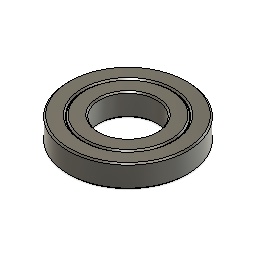
LR2051-822 (Autodesk Fusion 360 design; units mm, degrees)
Autodesk Fusion 360 part; units mm, degrees
sketch "profile" plane through (0, 0, 0) normal (0, 0, 1) x (1, 0, 0) in component "LR2051-822"
  line L0 (0, 0) -> (0, 8) construction
  line L1 (-10, 8) -> (-21, 8)
  line L2 (-21, 8) -> (-21, 0)
  line L3 (-21, 0) -> (-10, 0)
  line L4 (-10, 8) -> (-10, 0)
  line L5 (0, 8) -> (-10, 8) construction
  line L6 (-10, 0) -> (0, 0) construction
  line L7 (-15.5, 0) -> (-15.5, 1) construction
  line L8 (-15.5, 1) -> (-17, 2.5) construction
  line L9 (-17, 2.5) -> (-14, 5.5) construction
  line L10 (-14, 5.5) -> (-15.5, 7) construction
  line L11 (-15.5, 7) -> (-15.5, 8) construction
  line L12 (-10, 4) -> (-21, 4) construction
  line L13 (-15.5, 7) -> (-15.5, 1) construction
  line L14 (-15.4, 0) -> (-15.4, 1.0414)
  line L15 (-15.4, 1.0414) -> (-16.8586, 2.5)
  line L16 (-16.8586, 2.5) -> (-13.8586, 5.5)
  line L17 (-13.8586, 5.5) -> (-15.4, 7.0414)
  line L18 (-15.4, 7.0414) -> (-15.4, 8)
  line L19 (-15.6, 0) -> (-15.6, 0.9586)
  line L20 (-15.6, 0.9586) -> (-17.1414, 2.5)
  line L21 (-17.1414, 2.5) -> (-14.1414, 5.5)
  line L22 (-14.1414, 5.5) -> (-15.6, 6.9586)
  line L23 (-15.6, 6.9586) -> (-15.6, 8)
  point P0 (-15.5, 4)
  dimension "d4" = 21
  dimension "d5" = 10
  dimension "d6" = 45
  dimension "d7" = 1.5
  dimension "d8" = 1.5
  dimension "d9" = 8
  dimension "d10" = 0.1
  dimension "d11" = -0.1
  constraint coincident L0.start L6.end
  constraint vertical L0
  constraint perpendicular L0 L1
  constraint perpendicular L1 L2
  constraint perpendicular L0 L3
  constraint perpendicular L3 L4
  constraint perpendicular L0 L5
  constraint perpendicular L0 L6
  constraint midpoint L3 L7.start
  constraint perpendicular L3 L7
  constraint midpoint L1 L11.end
  constraint perpendicular L1 L11
  constraint midpoint L4 L12.start
  constraint midpoint L2 L12.end
  constraint parallel L8 L10
  constraint perpendicular L8 L9
  constraint midpoint L12 P0
  constraint coincident L9 P0
  measures "d4" distance of L2 L0.start
  measures "d5" distance of L0.start L4
  measures "d6" angle of L8 L13
  measures "d7" distance of L9.end L13
  measures "d8" distance of L8.end L11
  measures "d9" distance of L1.end L2.end
revolve "Revolve1" add sketch "profile" angle 360 about axis through (0, 0, 0) along (0, 1, 0) contours L1 L3 L4 L14 L15 L16 L17 L18 makes body 1 in component "Inner Shell"
revolve "Revolve1'" add sketch "profile" angle 360 about axis through (0, 0, 0) along (0, 1, 0) separate body contours L1 L2 L3 L19 L20 L21 L22 L23 makes body 2 in component "Outer Shell"
chamfer "Chamfer1" distance 0.5 angle 45 2 edges at (-14.3578, 8, 5.5689) (-14.3578, 0, 5.5689) on bodies 1 in component "Inner Shell"
chamfer "Chamfer2" distance 0.5 angle 45 2 edges at (-9.3233, 8, 3.6162) (-9.3233, 0, 3.6162) on bodies 1 in component "Inner Shell"
chamfer "Chamfer1'" distance 0.5 angle 45 2 edges at (-14.5443, 8, 5.6412) (-14.5443, 0, 5.6412) on bodies 2 in component "Outer Shell"
chamfer "Chamfer2'" distance 0.5 angle 45 2 edges at (-19.5789, 8, 7.5939) (-19.5789, 0, 7.5939) on bodies 2 in component "Outer Shell"
fillet "Fillet1" radius 0.5 2 edges at (-12.9207, 5.5, 5.0115) (-15.7177, 2.5, 6.0963) on bodies 1 in component "Inner Shell"
fillet "Fillet1'" radius 0.5 2 edges at (-13.1844, 5.5, 5.1138) (-15.9814, 2.5, 6.1986) on bodies 2 in component "Outer Shell"
component "LR2051-822" placed x (1, 0, 0) y (0, 1, 0) z (0, 0, 1) at (0, 0, 0)
component "Inner Shell" placed x (1, 0, 0) y (0, 1, 0) z (0, 0, 1) at (0, 0, 0) in component "LR2051-822"
component "Outer Shell" placed x (1, 0, 0) y (0, 1, 0) z (0, 0, 1) at (0, 0, 0) in component "LR2051-822"
equation "inner_dia = 20 mm"
equation "outer_dia = 42 mm"
equation "width = 8 mm"
equation "d4 = outer_dia / 2"
equation "d5 = inner_dia / 2"
equation "d8 = d7"
equation "d9 = width"
equation "d10 = gap / 2"
equation "d11 = -gap / 2"
equation "gap = 0.2 mm"
equation "outer_chamfer = 0.5 mm"
equation "inner_chamfer = 0.5 mm"
equation "d17 = inner_chamfer"
equation "d18 = outer_chamfer"
equation "d19 = inner_chamfer"
equation "d20 = outer_chamfer"
named bodies: "inner_shell", "outer_shell"
